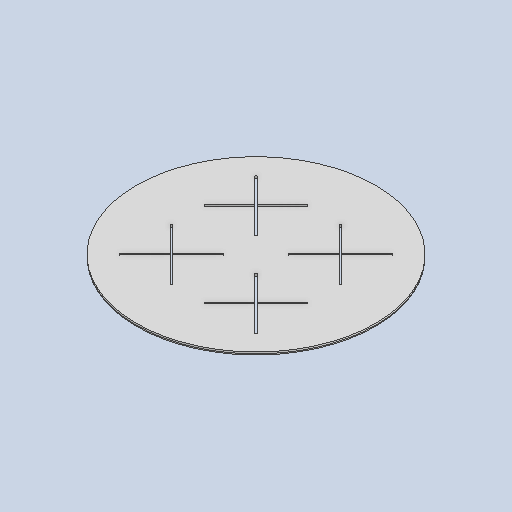
# Autodesk Inventor part: Sustainable Chair_V2 - Seat
Saved by Autodesk Inventor 2025.2 (Build 292293000, 293)
## iProperties
Created: 2025-02-10
Part Number: Sustainable Chair_V2 - Seat
Material: Foam Board - V3
Document SubType Name: Modeling
Designer: Dylan
Density: 0.151132 g/cm^3
Appearance: Default
Mass: 88.7045 g
Surface Area: 2615.45 cm^2
Volume: 586.933 cm^3
Author: Dylan
Autodesk Inventor part; units mm, degrees
ref_plane "YZ Plane" through (0, 0, 0) normal (1, 0, 0) x (0, 1, 0)
ref_plane "XZ Plane" through (0, 0, 0) normal (0, 1, 0) x (-1, 0, 0)
ref_plane "XY Plane" through (0, 0, 0) normal (0, 0, 1) x (1, 0, 0)
sketch "Sketch1" plane through (0, 0, 0) normal (0, 1, 0) x (-1, 0, 0)
  circle A0 centre (0, 0) radius 200
  dimension "d0" = 400
  constraints: 1 centre point, 1 coincident
  measures "d0" diameter of A0
extrude "Extrusion1" add sketch "Sketch1" along normal blind 4.7625
chamfer "Chamfer1" distance 2 angle 12.5 1 edges at (200, 0, 0) measured on face at (200, 0.5, 0)
sketch "Sketch2" plane through (0, 4.7625, 0) normal (0, 1, 0) x (1, 0, 0)
  line L0 (0, 0) -> (200, 0) construction
  line L1 (0, 0) -> (160, 0) construction
  line L2 (0, 0) -> (100, 0) construction
  line L3 (88.3859, -54.7142) -> (54.7142, -88.3859)
  line L4 (54.7142, -88.3859) -> (53.0355, -86.7072)
  line L5 (53.0355, -86.7072) -> (86.7072, -53.0355)
  line L6 (88.3859, -54.7142) -> (86.7072, -53.0355)
  line L7 (54.7142, -53.0355) -> (53.0355, -54.7142)
  line L8 (53.0355, -54.7142) -> (86.7072, -88.3859)
  line L9 (86.7072, -88.3859) -> (88.3859, -86.7072)
  line L10 (88.3859, -86.7072) -> (54.7142, -53.0355)
  circle A0 centre (0, 0) radius 200 projected
  line L11 (-88.3859, -54.7142) -> (-54.7142, -88.3859)
  line L12 (-54.7142, -88.3859) -> (-53.0355, -86.7072)
  line L13 (-53.0355, -86.7072) -> (-86.7072, -53.0355)
  line L14 (-88.3859, -54.7142) -> (-86.7072, -53.0355)
  line L15 (-54.7142, -53.0355) -> (-53.0355, -54.7142)
  line L16 (-53.0355, -54.7142) -> (-86.7072, -88.3859)
  line L17 (-86.7072, -88.3859) -> (-88.3859, -86.7072)
  line L18 (-88.3859, -86.7072) -> (-54.7142, -53.0355)
  line L19 (88.3859, 54.7142) -> (54.7142, 88.3859)
  line L20 (54.7142, 88.3859) -> (53.0355, 86.7072)
  line L21 (53.0355, 86.7072) -> (86.7072, 53.0355)
  line L22 (88.3859, 54.7142) -> (86.7072, 53.0355)
  line L23 (54.7142, 53.0355) -> (53.0355, 54.7142)
  line L24 (53.0355, 54.7142) -> (86.7072, 88.3859)
  line L25 (86.7072, 88.3859) -> (88.3859, 86.7072)
  line L26 (88.3859, 86.7072) -> (54.7142, 53.0355)
  line L27 (-88.3859, 54.7142) -> (-54.7142, 88.3859)
  line L28 (-54.7142, 88.3859) -> (-53.0355, 86.7072)
  line L29 (-53.0355, 86.7072) -> (-86.7072, 53.0355)
  line L30 (-53.0355, 54.7142) -> (-86.7072, 88.3859)
  line L31 (-88.3859, 86.7072) -> (-54.7142, 53.0355)
  line L32 (-86.7072, 88.3859) -> (-88.3859, 86.7072)
  line L33 (-88.3859, 54.7142) -> (-86.7072, 53.0355)
  line L34 (-54.7142, 53.0355) -> (-53.0355, 54.7142)
  point P0 (69.032, 70.7107)
  point P1 (70.7107, 69.032)
  point P2 (72.3893, 70.7107)
  point P3 (70.7107, 72.3893)
  point P4 (-69.032, 70.7107)
  point P5 (-70.7107, 72.3893)
  point P6 (-72.3893, 70.7107)
  point P7 (-70.7107, 69.032)
  point P8 (-72.3893, -70.7107)
  point P9 (-70.7107, -72.3893)
  point P10 (-69.032, -70.7107)
  point P11 (-70.7107, -69.032)
  point P12 (72.3893, -70.7107)
  point P13 (70.7107, -69.032)
  point P14 (69.032, -70.7107)
  point P15 (70.7107, -72.3893)
  dimension "d16" = 2.374
  dimension "d20" = 47.619
  constraints: 70 end point, 3 horizontal, 2 perpendicular, 1 horizontal alignment
  measures "d16" distance of L3.end L4.end
  measures "d20" distance of L7.end L8.end
extrude "Extrusion2" cut sketch "Sketch2" against normal blind 10 contours L3 L10 L5 L6 | L10 L9 L8 L3 | L3 L8 L5 L10 | L3 L4 L5 L8 | L5 L8 L7 L10 | L14 L13 L18 L11 | L18 L13 L16 L11 | L11 L16 L17 L18 | L16 L13 L12 L11 | L18 L15 L16 L13 | L22 L21 L26 L19 | L26 L21 L24 L19 | L19 L24 L25 L26 | L24 L21 L20 L19 | L26 L23 L24 L21 | L27 L31 L29 L33 | L31 L32 L30 L27 | L27 L30 L29 L31 | L27 L28 L29 L30 | L29 L30 L34 L31
sketch "Sketch3" plane through (0, 4.7625, 0) normal (0, 1, 0) x (1, 0, 0)
  line L0 (-54.7142, 53.0355) -> (-28.1977, 26.519)
  line L1 (-53.0355, 54.7142) -> (-26.519, 28.1977)
  line L2 (-26.519, 28.1977) -> (-28.1977, 26.519)
  line L3 (-53.0355, 54.7142) -> (-54.7142, 53.0355)
  line L4 (-88.3859, 86.7072) -> (-114.9024, 113.2237)
  line L5 (-86.7072, 88.3859) -> (-113.2237, 114.9024)
  line L6 (-113.2237, 114.9024) -> (-114.9024, 113.2237)
  line L7 (-86.7072, 88.3859) -> (-88.3859, 86.7072)
  line L8 (-54.7142, 88.3859) -> (-53.0355, 86.7072)
  line L9 (-53.0355, 86.7072) -> (-26.519, 113.2237)
  line L10 (-54.7142, 88.3859) -> (-28.1977, 114.9024)
  line L11 (-28.1977, 114.9024) -> (-26.519, 113.2237)
  line L12 (-88.3859, 54.7142) -> (-86.7072, 53.0355)
  line L13 (-86.7072, 53.0355) -> (-113.2237, 26.519)
  line L14 (-88.3859, 54.7142) -> (-114.9024, 28.1977)
  line L15 (-114.9024, 28.1977) -> (-113.2237, 26.519)
  circle A0 centre (0, 0) radius 200 projected
  line L16 (-54.7142, -53.0355) -> (-28.1977, -26.519)
  line L17 (-53.0355, -54.7142) -> (-26.519, -28.1977)
  line L18 (-26.519, -28.1977) -> (-28.1977, -26.519)
  line L19 (-53.0355, -54.7142) -> (-54.7142, -53.0355)
  line L20 (-86.7072, -88.3859) -> (-113.2237, -114.9024)
  line L21 (-86.7072, -88.3859) -> (-88.3859, -86.7072)
  line L22 (-88.3859, -86.7072) -> (-114.9024, -113.2237)
  line L23 (-113.2237, -114.9024) -> (-114.9024, -113.2237)
  line L24 (-54.7142, -88.3859) -> (-53.0355, -86.7072)
  line L25 (-53.0355, -86.7072) -> (-26.519, -113.2237)
  line L26 (-54.7142, -88.3859) -> (-28.1977, -114.9024)
  line L27 (-28.1977, -114.9024) -> (-26.519, -113.2237)
  line L28 (-114.9024, -28.1977) -> (-113.2237, -26.519)
  line L29 (-88.3859, -54.7142) -> (-114.9024, -28.1977)
  line L30 (-86.7072, -53.0355) -> (-113.2237, -26.519)
  line L31 (-88.3859, -54.7142) -> (-86.7072, -53.0355)
  line L32 (54.7142, 53.0355) -> (28.1977, 26.519)
  line L33 (53.0355, 54.7142) -> (26.519, 28.1977)
  line L34 (26.519, 28.1977) -> (28.1977, 26.519)
  line L35 (53.0355, 54.7142) -> (54.7142, 53.0355)
  line L36 (86.7072, 88.3859) -> (113.2237, 114.9024)
  line L37 (86.7072, 88.3859) -> (88.3859, 86.7072)
  line L38 (88.3859, 86.7072) -> (114.9024, 113.2237)
  line L39 (113.2237, 114.9024) -> (114.9024, 113.2237)
  line L40 (54.7142, 88.3859) -> (53.0355, 86.7072)
  line L41 (53.0355, 86.7072) -> (26.519, 113.2237)
  line L42 (54.7142, 88.3859) -> (28.1977, 114.9024)
  line L43 (28.1977, 114.9024) -> (26.519, 113.2237)
  line L44 (114.9024, 28.1977) -> (113.2237, 26.519)
  line L45 (88.3859, 54.7142) -> (114.9024, 28.1977)
  line L46 (86.7072, 53.0355) -> (113.2237, 26.519)
  line L47 (88.3859, 54.7142) -> (86.7072, 53.0355)
  line L48 (54.7142, -88.3859) -> (28.1977, -114.9024)
  line L49 (53.0355, -86.7072) -> (26.519, -113.2237)
  line L50 (54.7142, -88.3859) -> (53.0355, -86.7072)
  line L51 (28.1977, -114.9024) -> (26.519, -113.2237)
  line L52 (53.0355, -54.7142) -> (54.7142, -53.0355)
  line L53 (53.0355, -54.7142) -> (26.519, -28.1977)
  line L54 (54.7142, -53.0355) -> (28.1977, -26.519)
  line L55 (26.519, -28.1977) -> (28.1977, -26.519)
  line L56 (88.3859, -54.7142) -> (86.7072, -53.0355)
  line L57 (88.3859, -54.7142) -> (114.9024, -28.1977)
  line L58 (86.7072, -53.0355) -> (113.2237, -26.519)
  line L59 (114.9024, -28.1977) -> (113.2237, -26.519)
  line L60 (88.3859, -86.7072) -> (114.9024, -113.2237)
  line L61 (86.7072, -88.3859) -> (113.2237, -114.9024)
  line L62 (113.2237, -114.9024) -> (114.9024, -113.2237)
  line L63 (86.7072, -88.3859) -> (88.3859, -86.7072)
  constraints: 128 end point, 1 perpendicular
extrude "Extrusion3" cut sketch "Sketch3" against normal blind 10 contours L3 L1 L2 L0 | L4 L6 L5 L7 | L10 L11 L9 L8 | L12 L13 L15 L14 | L16 L18 L17 L19 | L20 L23 L22 L21 | L24 L25 L27 L26 | L28 L30 L31 L29 | L32 L34 L33 L35 | L36 L39 L38 L37 | L40 L41 L43 L42 | L44 L46 L47 L45 | L48 L51 L49 L50 | L53 L55 L54 L52 | L56 L58 L59 L57 | L60 L62 L61 L63
body "Solid1"
